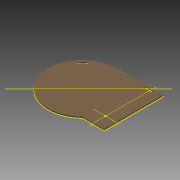
# Autodesk Inventor part: Base_Left
Saved by Autodesk Inventor 2014 SP1 (Build 180222100, 222)
## iProperties
Created: 2014-01-12
Part Number: Base_Left
Material: MDF Medium Density Fiberboard
Document SubType Name: Modeling
Designer: tuleu
Density: 0.8 g/cm^3
Appearance: Cardboard - Corrugated
Author: tuleu
Autodesk Inventor part; units mm, degrees
ref_plane "YZ Plane" through (0, 0, 0) normal (1, 0, 0) x (0, 1, 0)
ref_plane "XZ Plane" through (0, 0, 0) normal (0, 1, 0) x (-1, 0, 0)
ref_plane "XY Plane" through (0, 0, 0) normal (0, 0, 1) x (1, 0, 0)
sketch "Sketch1" plane through (0, 0, 0) normal (0, 1, 0) x (-1, 0, 0)
  arc A0 (0, -490) -> (-342.9286, 350) centre (0, 0) ccw
  line L0 (0, -490) -> (-650, -490)
  line L1 (-650, -490) -> (-650, 350)
  line L2 (-650, 350) -> (-342.9286, 350)
  dimension "d1" = 980
  dimension "d2" = 350
  dimension "d3" = 650
  constraints: 6 end point, 2 point on circle, 1 centre point, 1 coincident, 1 horizontal, 1 parallel, 1 perpendicular, 1 tangent
  measures "d1" diameter of A0
  measures "d2" distance from line of point (0, 0) L2
  measures "d3" distance from line of point (0, 0) L1
extrude "Extrusion1" add sketch "Sketch1" along normal mid plane 16
sketch "Sketch2" plane through (0, 8, 0) normal (0, 1, 0) x (1, 0, 0)
  arc A0 (0, 490) -> (342.9286, -350) centre (0, 0) ccw projected
  line L0 (650, -350) -> (650, 490) projected
  line L1 (650, 490) -> (0, 490) projected
  line L2 (435, 465) -> (525, 465)
  line L3 (530, 460) -> (530, 445)
  line L4 (525, 440) -> (435, 440)
  line L5 (430, 445) -> (430, 460)
  arc A1 (435, 465) -> (430, 460) centre (435, 460) ccw
  arc A2 (430, 445) -> (435, 440) centre (435, 445) ccw
  arc A3 (525, 440) -> (530, 445) centre (525, 445) ccw
  arc A4 (530, 460) -> (525, 465) centre (525, 460) ccw
  line L6 (0, 0) -> (-346.4823, 346.4823) construction
  line L7 (-289.9138, 353.5534) -> (-353.5534, 289.9138)
  line L8 (-353.5534, 282.8427) -> (-342.9468, 272.2361)
  line L9 (-335.8757, 272.2361) -> (-272.2361, 335.8757)
  line L10 (-272.2361, 342.9468) -> (-282.8427, 353.5534)
  arc A5 (-353.5534, 289.9138) -> (-353.5534, 282.8427) centre (-350.0179, 286.3782) ccw
  arc A6 (-342.9468, 272.2361) -> (-335.8757, 272.2361) centre (-339.4113, 275.7716) ccw
  arc A7 (-272.2361, 335.8757) -> (-272.2361, 342.9468) centre (-275.7716, 339.4113) ccw
  arc A8 (-282.8427, 353.5534) -> (-289.9138, 353.5534) centre (-286.3782, 350.0179) ccw
  point P0 (430, 465)
  point P1 (530, 465)
  point P2 (430, 440)
  dimension "d6" = 100
  dimension "d7" = 25
  dimension "d8" = 25
  dimension "d9" = 120
  dimension "d10" = 5
  dimension "d11" = 45
  dimension "d15" = 25
  dimension "d16" = 100
  dimension "d17" = 430
  dimension "d18" = 90
  dimension "d19" = 5
  constraints: 18 end point, 17 point on circle, 16 tangent, 8 centre point, 6 equal radius, 6 point on line, 4 parallel, 2 perpendicular, 1 horizontal, 1 other
  measures "d6" distance of point (430, 465) point (530, 465)
  measures "d7" distance of point (430, 440) point (430, 465)
  measures "d8" distance between parallel lines of L1 L2
  measures "d9" distance between parallel lines of L0 L3
  measures "d10" radius of A1
  measures "d11" angle of L0 L6
  measures "d15" distance between parallel lines of L9 L7
  measures "d16" distance between parallel lines of L8 L10
  measures "d17" distance from line of L6.start L9
  measures "d18" distance of L4.start L4.end
  measures "d19" radius of A5
extrude "Extrusion2" cut sketch "Sketch2" against normal through all
sketch "Sketch3" plane through (0, 8, 0) normal (0, 1, 0) x (1, 0, 0)
  circle A0 centre (610, 470) radius 4
  circle A1 centre (610, -330) radius 4
  circle A2 centre (610, 70) radius 4
  circle A3 centre (610, 470) radius 2.75 projected
  circle A4 centre (610, 70) radius 2.75 projected
  circle A5 centre (610, -330) radius 2.75 projected
  dimension "d22" = 8
  constraints: 3 centre point, 3 coincident, 2 equal radius
  measures "d22" diameter of A0
extrude "Extrusion3" cut sketch "Sketch3" against normal through all contours A0 | A1 | A2 | A3 | A4 | A5
ref_plane "Work Plane1" through (0, 0, 0) normal (-0.7071, 0, -0.7071) x (-0.7071, 0, 0.7071)
ref_plane "Work Plane2" through (500, 8, 350) normal (1, 0, 0) x (0, 0, -1)
ref_plane "Work Plane3" through (342.9286, 8, 180) normal (0, 0, 1) x (1, 0, 0)
sketch "Sketch5" plane through (0, -8, 0) normal (0, -1, 0) x (1, 0, 0)
  circle A0 centre (610, 330) radius 4 projected
  circle A1 centre (610, -470) radius 4 projected
  circle A2 centre (610, -70) radius 4 projected
  arc A3 (435, -440) -> (430, -445) centre (435, -445) ccw projected
  line L0 (435, -440) -> (525, -440) projected
  arc A4 (530, -445) -> (525, -440) centre (525, -445) ccw projected
  line L1 (530, -445) -> (530, -460) projected
  arc A5 (525, -465) -> (530, -460) centre (525, -460) ccw projected
  line L2 (525, -465) -> (435, -465) projected
  arc A6 (430, -460) -> (435, -465) centre (435, -460) ccw projected
  line L3 (430, -460) -> (430, -445) projected
  arc A7 (-335.8757, -272.2361) -> (-342.9468, -272.2361) centre (-339.4113, -275.7716) ccw projected
  line L4 (-335.8757, -272.2361) -> (-272.2361, -335.8757) projected
  arc A8 (-272.2361, -342.9468) -> (-272.2361, -335.8757) centre (-275.7716, -339.4113) ccw projected
  line L5 (-272.2361, -342.9468) -> (-282.8427, -353.5534) projected
  arc A9 (-289.9138, -353.5534) -> (-282.8427, -353.5534) centre (-286.3782, -350.0179) ccw projected
  line L6 (-289.9138, -353.5534) -> (-353.5534, -289.9138) projected
  arc A10 (-353.5534, -282.8427) -> (-353.5534, -289.9138) centre (-350.0179, -286.3782) ccw projected
  line L7 (-353.5534, -282.8427) -> (-342.9468, -272.2361) projected
  arc A11 (342.9286, 350) -> (0, -490) centre (0, 0) ccw projected
  line L8 (0, -490) -> (650, -490) projected
  line L9 (650, -490) -> (650, 350) projected
  line L10 (650, 350) -> (342.9286, 350) projected
  line L11 (0, 0) -> (650, 0) construction
  line L12 (0, 0) -> (0, -490) construction
  constraints: 4 end point, 2 perpendicular, 1 point on line
body "Solid1"
